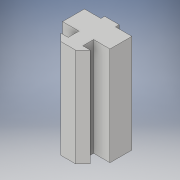
# Autodesk Inventor part: ppppaaaarrrrttttssss
Saved by Autodesk Inventor 2018 (Build 220112000, 112)
## iProperties
Created: 2019-12-04
Part Number: ppppaaaarrrrttttssss
Material: Generic
Document SubType Name: Modeling
Designer: AOFUser
Density: 1 g/cm^3
Appearance: Default
Author: AOFUser
Autodesk Inventor part; units mm, degrees
ref_plane "YZ Plane" through (0, 0, 0) normal (1, 0, 0) x (0, 1, 0)
ref_plane "XZ Plane" through (0, 0, 0) normal (0, 1, 0) x (-1, 0, 0)
ref_plane "XY Plane" through (0, 0, 0) normal (0, 0, 1) x (1, 0, 0)
sketch "Sketch1" plane through (0, 0, 0) normal (0, 1, 0) x (-1, 0, 0)
  line L0 (8.2818, 3.8463) -> (-8.2282, 3.8463)
  line L1 (-8.2282, 3.8463) -> (-8.2282, -3.7737)
  line L2 (-8.2282, -3.7737) -> (8.2818, -3.7737)
  line L3 (8.2818, -3.7737) -> (8.2818, 3.8463)
  line L4 (2.541, 10.1638) -> (-2.539, 10.1638)
  line L5 (-2.539, 10.1638) -> (-2.539, -5.0762)
  line L6 (-2.539, -5.0762) -> (2.541, -5.0762)
  line L7 (2.541, -5.0762) -> (2.541, 10.1638)
  line L8 (2.541, 7.6238) -> (5.081, 7.6238)
  line L9 (5.081, 7.6238) -> (2.541, 10.1638)
  line L10 (-2.539, 7.6238) -> (-5.079, 7.6238)
  line L11 (-5.079, 7.6238) -> (-2.539, 10.1638)
  dimension "d10" = 16.51
  dimension "d11" = 7.62
  dimension "d12" = 5.08
  dimension "d13" = 15.24
  dimension "d18" = 2.54
  dimension "d19" = 2.54
  constraints: 24 end point, 4 horizontal, 4 parallel, 2 perpendicular, 2 point on line
  measures "d10" distance of L2.end L1.end
  measures "d11" distance of L1.end L0.end
  measures "d12" distance of L6.end L5.end
  measures "d13" distance of L5.end L4.end
  measures "d18" distance of L8.start L8.end
  measures "d19" distance of L10.start L10.end
extrude "Extrusion1" add sketch "Sketch1" along normal blind 34.29
body "Solid1"
